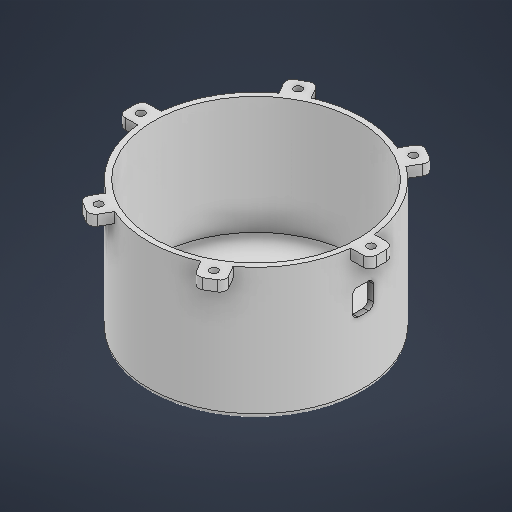
# Autodesk Inventor part: ruka base
Saved by Autodesk Inventor 2026 (Build 300175000, 175)
## iProperties
Created: 2025-04-11
Part Number: ruka base
Material: Generic
Document SubType Name: Modeling
Designer: janpa
Density: 1 g/cm^3
Appearance: Default
Author: janpa
Autodesk Inventor part; units mm, degrees
ref_plane "YZ Plane" through (0, 0, 0) normal (1, 0, 0) x (0, 1, 0)
ref_plane "XZ Plane" through (0, 0, 0) normal (0, 1, 0) x (-1, 0, 0)
ref_plane "XY Plane" through (0, 0, 0) normal (0, 0, 1) x (1, 0, 0)
sketch "Sketch1" plane through (0, 0, 0) normal (0, 1, 0) x (-1, 0, 0)
  circle A0 centre (0, 0) radius 41
  dimension "d0" = 82
  constraints: 1 centre point, 1 coincident
  measures "d0" diameter of A0
extrude "Extrusion1" add sketch "Sketch1" along normal blind 5.5
sketch "Sketch2" plane through (0, 5.5, 0) normal (0, 1, 0) x (1, 0, 0)
  circle A0 centre (0, 0) radius 41
  circle A1 centre (0, 0) radius 39
  circle A2 centre (0, 0) radius 6.75
  circle A3 centre (0, 0) radius 2.5
  dimension "d3" = 82
  dimension "d4" = 78
  dimension "d5" = 13.5
  dimension "d6" = 5
  constraints: 4 centre point, 4 coincident
  measures "d3" diameter of A0
  measures "d4" diameter of A1
  measures "d5" diameter of A2
  measures "d6" diameter of A3
extrude "Extrusion2" add sketch "Sketch2" along normal blind 45 contours A0
extrude "Extrusion3" cut sketch "Sketch2" along normal mid plane 45 contours A2 | A3
fillet "Fillet1" radius 2 1 edges at (41, 0, 0)
sketch "Sketch3" plane through (0, 50.5, 0) normal (0, 1, 0) x (1, 0, 0)
  line L0 (-40, -4.5) -> (-45.5, -4.5)
  line L1 (-48, -2) -> (-48, 2)
  line L2 (-45.5, 4.5) -> (-40, 4.5)
  line L3 (-40, 4.5) -> (-40, -4.5)
  circle A0 centre (-44, 0) radius 1.5
  circle A1 centre (-44, 0) radius 2.8
  arc A2 (-48, -2) -> (-45.5, -4.5) centre (-45.5, -2) ccw
  arc A3 (-45.5, 4.5) -> (-48, 2) centre (-45.5, 2) ccw
  line L4 (-57.15, -71.4375) -> (-33.3375, -71.4375)
  line L5 (-33.3375, -71.4375) -> (-33.3375, -57.15)
  line L6 (-23.8971, -32.391) -> (-16.1029, -36.891)
  line L7 (-16.1029, -36.891) -> (-18.8529, -41.6542)
  line L8 (-26.6471, -37.1542) -> (-23.8971, -32.391)
  circle A4 centre (-22, -38.1051) radius 1.5
  circle A5 centre (-22, -38.1051) radius 2.8
  line L9 (-22.2679, -42.5692) -> (-25.7321, -40.5692)
  arc A6 (-26.6471, -37.1542) -> (-25.7321, -40.5692) centre (-24.4821, -38.4042) ccw
  arc A7 (-22.2679, -42.5692) -> (-18.8529, -41.6542) centre (-21.0179, -40.4042) ccw
  line L10 (16.1029, -36.891) -> (23.8971, -32.391)
  line L11 (23.8971, -32.391) -> (26.6471, -37.1542)
  line L12 (18.8529, -41.6542) -> (16.1029, -36.891)
  circle A8 centre (22, -38.1051) radius 1.5
  circle A9 centre (22, -38.1051) radius 2.8
  line L13 (25.7321, -40.5692) -> (22.2679, -42.5692)
  arc A10 (18.8529, -41.6542) -> (22.2679, -42.5692) centre (21.0179, -40.4042) ccw
  arc A11 (25.7321, -40.5692) -> (26.6471, -37.1542) centre (24.4821, -38.4042) ccw
  line L14 (40, -4.5) -> (40, 4.5)
  line L15 (40, 4.5) -> (45.5, 4.5)
  line L16 (45.5, -4.5) -> (40, -4.5)
  circle A12 centre (44, 0) radius 1.5
  circle A13 centre (44, 0) radius 2.8
  line L17 (48, 2) -> (48, -2)
  arc A14 (45.5, -4.5) -> (48, -2) centre (45.5, -2) ccw
  arc A15 (48, 2) -> (45.5, 4.5) centre (45.5, 2) ccw
  line L18 (23.8971, 32.391) -> (16.1029, 36.891)
  line L19 (16.1029, 36.891) -> (18.8529, 41.6542)
  line L20 (26.6471, 37.1542) -> (23.8971, 32.391)
  circle A16 centre (22, 38.1051) radius 1.5
  circle A17 centre (22, 38.1051) radius 2.8
  line L21 (22.2679, 42.5692) -> (25.7321, 40.5692)
  arc A18 (26.6471, 37.1542) -> (25.7321, 40.5692) centre (24.4821, 38.4042) ccw
  arc A19 (22.2679, 42.5692) -> (18.8529, 41.6542) centre (21.0179, 40.4042) ccw
  line L22 (-16.1029, 36.891) -> (-23.8971, 32.391)
  line L23 (-23.8971, 32.391) -> (-26.6471, 37.1542)
  line L24 (-18.8529, 41.6542) -> (-16.1029, 36.891)
  circle A20 centre (-22, 38.1051) radius 1.5
  circle A21 centre (-22, 38.1051) radius 2.8
  line L25 (-25.7321, 40.5692) -> (-22.2679, 42.5692)
  arc A22 (-18.8529, 41.6542) -> (-22.2679, 42.5692) centre (-21.0179, 40.4042) ccw
  arc A23 (-25.7321, 40.5692) -> (-26.6471, 37.1542) centre (-24.4821, 38.4042) ccw
  point P0 (0, 0)
  point P1 (-48, 4.5)
  point P2 (-48, -4.5)
  point P3 (-20.1029, -43.8192)
  point P4 (-27.8971, -39.3192)
  point P5 (27.8971, -39.3192)
  point P6 (20.1029, -43.8192)
  point P7 (48, 4.5)
  point P8 (48, -4.5)
  point P9 (20.1029, 43.8192)
  point P10 (27.8971, 39.3192)
  point P11 (-27.8971, 39.3192)
  point P12 (-20.1029, 43.8192)
  dimension "d12" = 8
  dimension "d13" = 9
  dimension "d14" = 4.5
  dimension "d15" = 40
  dimension "d16" = 3
  dimension "d17" = 5.6
  dimension "d18" = 2.5
  dimension "d19" = 4
  dimension "d22" = 360
  constraints: 52 end point, 24 centre point, 24 point on circle, 24 point on line, 6 coincident, 4 tangent, 2 horizontal, 2 parallel, 2 perpendicular, 1 equal radius, 121 other
  measures "d12" distance of point (-48, 4.5) L2.end
  measures "d13" distance of point (-48, -4.5) point (-48, 4.5)
  measures "d14" distance from line of point (0, 0) L2
  measures "d15" distance from line of point (0, 0) L3
  measures "d16" diameter of A0
  measures "d17" diameter of A1
  measures "d18" radius of A2
  measures "d19" distance from line of L3 A1.centre
extrude "Extrusion4" add sketch "Sketch3" against normal blind 4 contours L0 A2 L1 A3 L2 L3 | A1 | L6 L7 A7 L9 A6 L8 | A5 | L10 L11 A11 L13 A10 L12 | A9 | L14 L15 A15 L17 A14 L16 | A13 | L18 L19 A19 L21 A18 L20 | A17 | L22 L23 A23 L25 A22 L24 | A21
sketch "Sketch4" plane through (0, 46.5, 0) normal (0, -1, 0) x (1, 0, 0)
  circle A0 centre (-22, 38.1051) radius 1.5 projected
  circle A1 centre (-22, 38.1051) radius 2.75
  circle A2 centre (-44, 0) radius 2.75
  circle A3 centre (-22, -38.1051) radius 2.75
  circle A4 centre (22, -38.1051) radius 2.75
  circle A5 centre (44, 0) radius 2.75
  circle A6 centre (22, 38.1051) radius 2.75
  point P0 (0, 0)
  dimension "d26" = 5.5
  dimension "d29" = 360
  constraints: 6 centre point, 1 coincident, 13 other
  measures "d26" diameter of A1
extrude "Extrusion5" cut sketch "Sketch4" against normal blind 1
sketch "Sketch7" plane through (48, 50.5, 2) normal (1, 0, 0) x (0, 0, -1)
  line L0 (6, -24) -> (-2, -24)
  line L1 (-2, -24) -> (-2, -14)
  line L2 (-2, -14) -> (6, -14)
  line L3 (6, -14) -> (6, -24)
  line L4 (4, -4) -> (0, -4) projected
  line L5 (6.5, 0) -> (6.5, -4) projected
  line L6 (-2.5, 0) -> (-2.5, -4) projected
  point P0 (2, -50.5)
  point P1 (2, -14)
  dimension "d57" = 10
  dimension "d58" = 10
  dimension "d59" = 8
  dimension "d64" = 0.5
  constraints: 8 end point, 2 parallel, 1 horizontal, 1 midpoint, 1 perpendicular
  measures "d57" distance from line of L4 point (2, -14)
  measures "d58" distance of L2.end L0.start
  measures "d59" distance of L0.start L0.end
  measures "d64" distance between parallel lines of L5 L3
extrude "Extrusion8" cut sketch "Sketch7" against normal blind 50
fillet "Fillet2" radius 2 4 edges at (39.7994, 26.5, 4) (39.7994, 26.5, -4) (39.7994, 36.5, 4) (39.7994, 36.5, -4)
sketch "Sketch8" plane through (0, 5.5, 0) normal (0, 1, 0) x (1, 0, 0)
  line L0 (-4.75, 16.5) -> (4.75, 16.5)
  line L1 (4.75, 16.5) -> (4.75, -33.1)
  line L2 (4.75, -33.1) -> (-4.75, -33.1)
  line L3 (-4.75, -33.1) -> (-4.75, 16.5)
  line L4 (0, 64.4352) -> (0, -70.5607)
  circle A0 centre (-4.75, 16.5) radius 1.9
  circle A1 centre (4.75, 16.5) radius 1.9
  circle A2 centre (-4.75, -33.1) radius 1.9
  circle A3 centre (4.75, -33.1) radius 1.9
  point P0 (0, 0)
  point P1 (0, 16.5)
  dimension "d70" = 9.5
  dimension "d71" = 49.6
  dimension "d73" = 33
  dimension "d74" = 3.8
  constraints: 10 end point, 4 centre point, 4 coincident, 2 parallel, 2 point on line, 1 horizontal, 1 midpoint, 1 perpendicular, 1 vertical
  measures "d70" distance of L1.end L2.end
  measures "d71" distance of L0.end L1.end
  measures "d73" diameter of point (0, 0) L0
  measures "d74" diameter of A0
extrude "Extrusion10" cut sketch "Sketch8" against normal blind 5.1 contours L3 A0 L0 | L0 A0 L3 | A2 L2 L3 | L3 L2 A2 | A1 L1 L0 | L0 L1 A1 | A3 L1 L2 | L2 L1 A3
body "Solid1"
